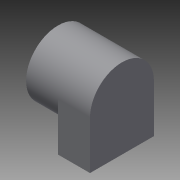
# Autodesk Inventor part: uchwytG5
Saved by Autodesk Inventor 2014 (Build 180170000, 170)
## iProperties
Created: 2013-12-25
Part Number: uchwytG5
Material: Ogólny
Document SubType Name: Modeling
Designer: Kuba
Density: 1 g/cm^3
Appearance: Domyślna
Author: Kuba
Autodesk Inventor part; units mm, degrees
ref_plane "YZ Plane" through (0, 0, 0) normal (1, 0, 0) x (0, 1, 0)
ref_plane "XZ Plane" through (0, 0, 0) normal (0, 1, 0) x (-1, 0, 0)
ref_plane "XY Plane" through (0, 0, 0) normal (0, 0, 1) x (1, 0, 0)
sketch "Szkic1" plane through (0, 0, 0) normal (1, 0, 0) x (0, 1, 0)
  circle A0 centre (0, 0) radius 10
  line L0 (-14, 0) -> (14, 0) projected
  line L1 (0, -20) -> (0, 15) projected
  line L2 (10, 0) -> (10, -15)
  line L3 (-10, -15) -> (10, -15)
  line L4 (-10, 0) -> (-10, -15)
  dimension "d0" = 20
  dimension "d3" = 15
  constraints: 6 end point, 2 parallel, 2 point on line, 2 tangent, 1 centre point, 1 coincident, 1 perpendicular
  measures "d0" diameter of A0
  measures "d3" distance of L2.start L2.end
extrude "Wyciągnięcie proste2" add sketch "Szkic1" along normal blind 10
extrude "Wyciągnięcie proste3" add sketch "Szkic1" against normal blind 10 contours L0 L1 A0 | A0 L1 L0 | L1 L0 A0 | A0 L0 L1
